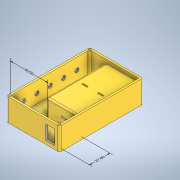
# Autodesk Inventor part: inferior model2
Saved by Autodesk Inventor 2020 (Build 240168000, 168)
## iProperties
Created: 2022-05-31
Part Number: inferior model2
Material: Generic
Document SubType Name: Modeling
Designer: juanc
Density: 1 g/cm^3
Appearance: Default
Author: juanc
Autodesk Inventor part; units mm, degrees
ref_plane "YZ Plane" through (0, 0, 0) normal (1, 0, 0) x (0, 1, 0)
ref_plane "XZ Plane" through (0, 0, 0) normal (0, 1, 0) x (-1, 0, 0)
ref_plane "XY Plane" through (0, 0, 0) normal (0, 0, 1) x (1, 0, 0)
sketch "Sketch1" plane through (0, 0, 0) normal (0, 1, 0) x (-1, 0, 0)
  line L0 (0, 0) -> (70, 0)
  line L1 (70, 0) -> (70, -110)
  line L2 (70, -110) -> (0, -110)
  line L3 (0, -110) -> (0, 0)
  line L4 (2.5, -2.5) -> (67.5, -2.5)
  line L5 (67.5, -2.5) -> (67.5, -107.5)
  line L6 (67.5, -107.5) -> (2.5, -107.5)
  line L7 (2.5, -107.5) -> (2.5, -2.5)
  line L8 (2.5, -2.5) -> (67.5, -107.5) construction
  line L9 (67.5, -2.5) -> (2.5, -107.5) construction
  point P0 (35, -55)
  dimension "d0" = 70
  dimension "d1" = 110
  dimension "d2" = 65
  dimension "d3" = 105
  constraints: 20 end point, 4 parallel, 2 horizontal, 2 midpoint, 2 perpendicular
  measures "d0" distance of L1.end L2.end
  measures "d1" distance of L0.end L1.end
  measures "d2" distance of L5.end L6.end
  measures "d3" distance of L4.end L5.end
extrude "Extrusion1" add sketch "Sketch1" along normal blind 30
sketch "Sketch2" plane through (0, 0, 0) normal (0, -1, 0) x (1, 0, 0)
  line L0 (0, -110) -> (-70, -110) projected
  line L1 (0, 0) -> (-70, 0)
  line L2 (-70, 0) -> (-70, -110)
  line L3 (-70, -110) -> (0, -110)
  line L4 (0, -110) -> (0, 0)
  constraints: 8 end point, 2 parallel, 1 horizontal, 1 perpendicular
extrude "Extrusion2" add sketch "Sketch2" against normal blind 3
sketch "Sketch3" plane through (0, 0, 0) normal (0, -1, 0) x (1, 0, 0)
  line L0 (-2.5, -107.5) -> (-2.5, -2.5) projected
  line L1 (-2.5, -107.5) -> (-46.5, -107.5)
  line L2 (-46.5, -107.5) -> (-46.5, -29.5)
  line L3 (-46.5, -29.5) -> (-2.5, -29.5)
  line L4 (-2.5, -29.5) -> (-2.5, -107.5)
  line L5 (-45.25, -106.5) -> (-3.75, -106.5)
  line L6 (-3.75, -106.5) -> (-3.75, -30.5)
  line L7 (-3.75, -30.5) -> (-45.25, -30.5)
  line L8 (-45.25, -30.5) -> (-45.25, -106.5)
  line L9 (-45.25, -106.5) -> (-3.75, -30.5) construction
  line L10 (-3.75, -106.5) -> (-45.25, -30.5) construction
  point P0 (0, 0)
  point P1 (-24.5, -68.5)
  dimension "d8" = 44
  dimension "d9" = 78
  dimension "d10" = 41.5
  dimension "d11" = 76
  constraints: 20 end point, 4 parallel, 2 horizontal, 2 midpoint, 2 perpendicular
  measures "d8" distance of L2.end L3.end
  measures "d9" distance of L1.end L2.end
  measures "d10" distance of L7.end L6.end
  measures "d11" distance of L6.end L5.end
extrude "Extrusion3" add sketch "Sketch3" against normal blind 25
extrude "Extrusion4" cut sketch "Sketch3" against normal blind 25 contours L8 L7 L6 L5
sketch "Sketch4" plane through (0, 25, 0) normal (0, 1, 0) x (1, 0, 0)
  line L0 (-46.5, 107.5) -> (-46.5, 29.5) projected
  line L1 (-2.5, 107.5) -> (-2.5, 29.5) projected
  line L2 (-46.5, 29.5) -> (-2.5, 29.5)
  line L3 (-2.5, 29.5) -> (-2.5, 107.5)
  line L4 (-2.5, 107.5) -> (-46.5, 107.5)
  line L5 (-46.5, 107.5) -> (-46.5, 29.5)
  point P0 (0, 0)
  point P1 (-2.5, 29.5)
  constraints: 8 end point, 2 parallel, 1 horizontal, 1 perpendicular
extrude "Extrusion5" add sketch "Sketch4" against normal blind 2
fillet "Fillet1" radius 2 3 edges at (-46.5, 25, -68.5) (-46.5, 14, -29.5) (-24.5, 25, -29.5)
sketch "Sketch5" plane through (0, 23, 0) normal (0, -1, 0) x (1, 0, 0)
  line L0 (-45.25, -30.5) -> (-3.75, -30.5) construction
  line L1 (-3.75, -30.5) -> (-3.75, -106.5) construction
  line L2 (-45.25, -30.5) -> (-3.75, -106.5) construction
  line L3 (-3.75, -106.5) -> (-45.25, -106.5) construction
  line L4 (0, 0) -> (0, -110) construction
  line L5 (-45.25, -106.5) -> (-3.75, -30.5) construction
  line L6 (-24.5, -68.5) -> (-24.5, -106.5) construction
  line L7 (-3.75, -106.5) -> (-45.25, -106.5) construction
  line L8 (-24.5, -68.5) -> (-24.5, -30.5) construction
  line L9 (-45.25, -106.5) -> (-24.5, -30.5) construction
  line L10 (-45.25, -30.5) -> (-24.5, -106.5) construction
  line L11 (-24.5, -106.5) -> (-3.75, -30.5) construction
  line L12 (-24.5, -30.5) -> (-3.75, -106.5) construction
  line L13 (-31.875, -68.5) -> (-37.875, -68.5) construction
  line L14 (-31.875, -67.75) -> (-37.875, -67.75)
  line L15 (-37.875, -69.25) -> (-31.875, -69.25)
  arc A0 (-31.875, -69.25) -> (-31.875, -67.75) centre (-31.875, -68.5) ccw
  arc A1 (-37.875, -67.75) -> (-37.875, -69.25) centre (-37.875, -68.5) ccw
  line L16 (-11.125, -68.5) -> (-17.125, -68.5) construction
  line L17 (-11.125, -67.75) -> (-17.125, -67.75)
  line L18 (-17.125, -69.25) -> (-11.125, -69.25)
  arc A2 (-11.125, -69.25) -> (-11.125, -67.75) centre (-11.125, -68.5) ccw
  arc A3 (-17.125, -67.75) -> (-17.125, -69.25) centre (-17.125, -68.5) ccw
  point P0 (-34.875, -68.5)
  point P1 (-14.125, -68.5)
  dimension "d19" = 3
  dimension "d20" = 1.5
  dimension "d21" = 3
  dimension "d22" = 1.5
  constraints: 34 end point, 8 point on circle, 8 tangent, 7 midpoint, 4 centre point, 4 parallel, 2 horizontal, 1 perpendicular
  measures "d19" distance of point (-34.875, -68.5) L13.end
  measures "d20" diameter of A1
  measures "d21" distance of point (-14.125, -68.5) L16.end
  measures "d22" diameter of A3
extrude "Extrusion6" cut sketch "Sketch5" against normal blind 2
sketch "Sketch6" plane through (-44.5, 23, -29.5) normal (0, 0, 1) x (1, 0, 0)
  line L0 (44.5, 7) -> (44.5, -23) projected
  line L1 (44.5, -23) -> (-25.5, -23) projected
  line L2 (-25.5, -23) -> (-25.5, 7) projected
  line L3 (-25.5, 7) -> (-23, 7) projected
  line L4 (-23, 7) -> (-23, -20) projected
  line L5 (-23, -20) -> (0, -20) projected
  line L6 (0, -20) -> (0, 0) projected
  line L7 (0, 0) -> (42, 0) projected
  line L8 (42, -20) -> (42, 0) projected
  line L9 (0, -20) -> (42, -20) projected
  line L10 (42, 7) -> (44.5, 7) projected
  line L11 (42, 0) -> (42, 7) projected
  line L12 (42, 0) -> (0, -20) construction
  line L13 (42, -20) -> (0, 0) construction
  line L14 (18, -10) -> (24, -10) construction
  line L15 (18, -11) -> (24, -11)
  line L16 (24, -9) -> (18, -9)
  arc A0 (18, -9) -> (18, -11) centre (18, -10) ccw
  arc A1 (24, -11) -> (24, -9) centre (24, -10) ccw
  point P0 (21, -10)
  dimension "d25" = 3
  dimension "d26" = 2
  constraints: 12 end point, 4 point on circle, 4 tangent, 2 centre point, 2 midpoint, 1 horizontal, 1 parallel
  measures "d25" distance of point (21, -10) L14.end
  measures "d26" diameter of A1
extrude "Extrusion7" cut sketch "Sketch6" against normal blind 2 contours A0 L16 A1 L15
sketch "Sketch7" plane through (0, 30, 0) normal (0, 1, 0) x (1, 0, 0)
  line L0 (-67.5, 107.5) -> (-46.5, 107.5) projected
  circle A0 centre (-67.5, 107.5) radius 2.5
  line L1 (0, 110) -> (-70, 110) projected
  line L2 (-2.5, 2.5) -> (-67.5, 2.5) projected
  circle A1 centre (-2.5, 2.5) radius 2.5
  line L3 (-70, 0) -> (0, 0) projected
  circle A2 centre (-67.5, 2.5) radius 2.5
  constraints: 3 centre point, 3 tangent, 1 coincident
extrude "Extrusion8" add sketch "Sketch7" against normal blind 30 contours A0 | A1 | A2
fillet "Fillet2" radius 2 3 edges at (0, 15, 0) (-70, 15, 0) (-70, 15, -110)
sketch "Sketch8" plane through (0, 30, 0) normal (0, 1, 0) x (1, 0, 0)
  arc A0 (-65, 2.5) -> (-67.5, 5) centre (-67.5, 2.5) ccw projected
  arc A1 (-2.5, 5) -> (-5, 2.5) centre (-2.5, 2.5) ccw projected
  arc A2 (-67.5, 105) -> (-65, 107.5) centre (-67.5, 107.5) ccw projected
  point P0 (0, 0)
  constraints: 3 coincident
hole "Hole1" at (-67.5, 30, -2.5) at (-2.5, 30, -2.5) at (-67.5, 30, -107.5) direction (0, -1, 0) diameter 3 depth 40 tip angle 118
fillet "Fillet3" radius 2 1 edges at (0, 15, -110)
sketch "Sketch9" plane through (-45.25, 0, -106.5) normal (0, 0, 1) x (1, 0, 0)
  line L0 (-24.75, 30) -> (-23.368, 30) projected
  line L1 (-23.368, 30) -> (-23.368, 0) projected
  line L2 (-23.368, 0) -> (-24.75, 0) projected
  line L3 (-24.75, 0) -> (-24.75, 30) projected
  line L4 (41.5, 23) -> (0, 23) projected
  line L5 (0, 23) -> (0, 0) projected
  line L6 (0, 0) -> (-21.132, 0) projected
  line L7 (-21.132, 0) -> (-21.132, 30) projected
  line L8 (-21.132, 30) -> (-19.9587, 30) projected
  line L9 (-19.9587, 30) -> (-19.9587, 3) projected
  line L10 (-19.9587, 3) -> (-1.25, 3) projected
  line L11 (-1.25, 3) -> (-1.25, 23) projected
  arc A0 (0.75, 25) -> (-1.25, 23) centre (0.75, 23) ccw projected
  line L12 (0.75, 25) -> (42.75, 25) projected
  line L13 (42.75, 25) -> (42.75, 30) projected
  line L14 (42.75, 30) -> (45.25, 30) projected
  line L15 (45.25, 30) -> (45.25, 0) projected
  line L16 (45.25, 0) -> (41.5, 0) projected
  line L17 (41.5, 0) -> (0, 0) projected
  line L18 (41.5, 0) -> (41.5, 23) projected
  line L19 (0, 3) -> (2, 3) construction
  line L20 (-19.75, 3) -> (-1.25, 3) construction
  line L21 (2, 3) -> (4, 3)
  line L22 (4, 3) -> (4, 1)
  line L23 (4, 1) -> (2, 1)
  line L24 (2, 1) -> (2, 3)
  line L25 (41.5, 3) -> (39.5, 3) construction
  line L26 (39.5, 3) -> (37.5, 3)
  line L27 (37.5, 3) -> (37.5, 1)
  line L28 (37.5, 1) -> (39.5, 1)
  line L29 (39.5, 1) -> (39.5, 3)
  dimension "d40" = 2
  dimension "d41" = 2
  dimension "d42" = 2
  dimension "d43" = 2
  dimension "d44" = 2
  dimension "d45" = 2
  constraints: 20 end point, 4 parallel, 3 point on line, 2 horizontal, 2 perpendicular, 1 collinear
  measures "d40" distance of L19.start L19.end
  measures "d41" distance of L22.end L23.end
  measures "d42" distance of L21.end L22.end
  measures "d43" distance of L25.start L25.end
  measures "d44" distance of L28.end L27.end
  measures "d45" distance of L27.end L26.end
extrude "Extrusion9" cut sketch "Sketch9" against normal blind 2 contours L21 L22 L23 L24 | L29 L28 L27 L26
sketch "Sketch10" plane through (0, 0, 0) normal (0, -1, 0) x (1, 0, 0)
  line L0 (-45.25, -30.5) -> (-3.75, -30.5) projected
  circle A0 centre (-24.5, -30.5) radius 7.5
  point P0 (0, 0)
  point P1 (-17, -30.5)
  point P2 (-32, -30.5)
  dimension "d48" = 15
  constraints: 1 centre point, 1 midpoint
  measures "d48" diameter of A0
extrude "Extrusion10" cut sketch "Sketch10" against normal blind 1.5 contours A0 L0 picked at (-23.8998, -27.0007)
sketch "Sketch12" plane through (0, 1.5, 0) normal (0, -1, 0) x (1, 0, 0)
  arc A0 (-17, -30.5) -> (-32, -30.5) centre (-24.5, -30.5) ccw construction
  line L0 (-24.5, -30.5) -> (-24.5, -26.75) construction
  line L1 (-24.5, -30.5) -> (-20.75, -30.5) construction
  point P0 (0, 0)
  dimension "d58" = 3.75
  dimension "d59" = 90
  constraints: 4 end point, 1 coincident, 1 horizontal, 1 perpendicular, 1 vertical
  measures "d58" distance of L0.start L0.end
  measures "d59" angle of L1 L0
hole "Hole3" at (-24.5, 1.5, -26.75) direction (0, 1, 0) diameter 1 depth 1 tip angle 118
sketch "Sketch14" plane through (-70, 0, -108) normal (-1, 0, 0) x (0, 0, 1)
  line L0 (0, 0) -> (0, 30) construction
  line L1 (108, 0) -> (106, 0) construction
  line L2 (106, 0) -> (106, 30) construction
  line L3 (108, 30) -> (108, 0) construction
  line L4 (53, 15) -> (106, 15) construction
  line L5 (106, 0) -> (106, 30) construction
  line L6 (53, 15) -> (0, 15) construction
  line L7 (0, 15) -> (17.6, 15) construction
  point P0 (35.2, 15)
  point P1 (52.8, 15)
  point P2 (70.4, 15)
  point P3 (88, 15)
  dimension "d71" = 17.6
  dimension "d74" = 17.6
  dimension "d79" = 18
  constraints: 8 end point, 2 midpoint, 1 coincident, 1 horizontal, 1 parallel, 1 point on line, 4 other
  measures "d71" distance of L6.end L7.end
  measures "d74" distance of point (17.6, 15) point (35.2, 15)
  measures "d79" distance from line of L2 point (88, 15)
hole "Hole4" at (-70, 15, -90.4) at (-70, 15, -72.8) at (-70, 15, -55.2) at (-70, 15, -37.6) at (-70, 15, -20) direction (1, 0, 0) diameter 5.5 depth 3
sketch "Sketch16" plane through (-68, 0, 0) normal (0, 0, 1) x (1, 0, 0)
  line L0 (0, 0) -> (66, 0) construction
  line L1 (66, 0) -> (62, 0) construction
  line L2 (66, 0) -> (70, 0) construction
  line L3 (62, 0) -> (62, 30) construction
  line L4 (0, 30) -> (66, 30) construction
  line L5 (62, 23.7699) -> (50, 23.7699)
  line L6 (50, 23.7699) -> (50, 4.7699)
  line L7 (50, 4.7699) -> (62, 4.7699)
  line L8 (62, 4.7699) -> (62, 23.7699)
  point P0 (68, 0)
  dimension "d88" = 4
  dimension "d89" = 180
  dimension "d90" = 12
  dimension "d91" = 19
  constraints: 14 end point, 2 collinear, 2 horizontal, 2 parallel, 2 perpendicular, 2 point on line
  measures "d88" distance of L0.end L1.end
  measures "d89" angle of L1 L2
  measures "d90" distance of L7.end L6.end
  measures "d91" distance of L6.end L5.end
extrude "Extrusion11" cut sketch "Sketch16" against normal blind 3
body "Solid1"
